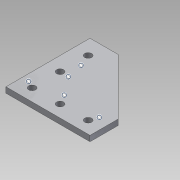
# Autodesk Inventor part: 5 Hole 90 Degree Bracket
Saved by Autodesk Inventor 2013 SP2 (Build 170200200, 200)
## iProperties
Created: 2013-07-08
Part Number: 5 Hole 90 Degree Bracket
Material: Aluminum 6061
Document SubType Name: Modeling
Designer: Jon Hollander
Density: 2.71 g/cm^3
Mass: 29.2878 g
Surface Area: 65.8408 cm^2
Volume: 10.8073 cm^3
Author: Jon Hollander
Autodesk Inventor part; units mm, degrees
ref_plane "YZ Plane" through (0, 0, 0) normal (1, 0, 0) x (0, 1, 0)
ref_plane "XZ Plane" through (0, 0, 0) normal (0, 1, 0) x (-1, 0, 0)
ref_plane "XY Plane" through (0, 0, 0) normal (0, 0, 1) x (1, 0, 0)
sketch "Sketch1" plane through (0, 0, 0) normal (0, 0, 1) x (1, 0, 0)
  line L0 (0, 0) -> (0, 60)
  line L1 (0, 0) -> (60, 0) construction
  line L2 (0, 60) -> (20, 60)
  line L3 (20, 60) -> (60, 20)
  line L4 (60, 20) -> (60, 0)
  line L5 (60, 0) -> (0, 0)
  point P0 (10, 8.6725)
  point P1 (30, 8.6725)
  point P2 (50, 8.6725)
  point P3 (10, 28.6725)
  point P4 (10, 48.6725)
  dimension "d0" = 60
  dimension "d1" = 90
  dimension "d2" = 20
  dimension "d3" = 135
  dimension "d4" = 60
  dimension "d5" = 20
  dimension "d6" = 10
  dimension "d7" = 20
  dimension "d8" = 20
  dimension "d9" = 20
  dimension "d10" = 20
  constraints: 12 end point, 2 parallel, 2 perpendicular, 2 vertical alignment, 1 horizontal, 1 vertical
  measures "d0" distance of L0.start L0.end
  measures "d1" angle of L1 L0
  measures "d2" distance of L0.end L2.end
  measures "d3" angle of L2 L3
  measures "d4" distance of L4.end L0.start
  measures "d5" distance of L3.end L4.end
  measures "d6" distance from line of L0 point (10, 8.673)
  measures "d7" distance of point (30, 8.673) point (10, 8.673)
  measures "d8" distance of point (50, 8.673) point (30, 8.673)
  measures "d9" distance of point (10, 28.673) point (10, 8.673)
  measures "d10" distance of point (10, 28.673) point (10, 48.673)
extrude "Extrusion1" add sketch "Sketch1" along normal blind 4
hole "Hole1" at (10, 8.6725, 0) at (30, 8.6725, 0) at (50, 8.6725, 0) at (10, 28.6725, 0) at (10, 48.6725, 0) direction (0, 0, 1) diameter 5 end through all
body "Solid1"
